Autodesk Inventor part; units mm, degrees
(part 3 of 13)
  spline S310 degree 3 poles (18.4407, 13.1537) (18.4407, 12.6177) (18.8752, 12.1831) (19.4112, 12.1831) knots 0 0 0 0 1 1 1 1
  line L939 (18.4407, 13.1537) -> (18.4407, 12.6177) construction
  line L940 (18.4407, 12.6177) -> (18.8752, 12.1831) construction
  line L941 (18.8752, 12.1831) -> (19.4112, 12.1831) construction
  spline S311 degree 3 poles (19.4112, 12.1831) (19.9472, 12.1831) (20.3818, 12.6177) (20.3818, 13.1537) knots 0 0 0 0 1 1 1 1
  line L942 (19.4112, 12.1831) -> (19.9472, 12.1831) construction
  line L943 (19.9472, 12.1831) -> (20.3818, 12.6177) construction
  line L944 (20.3818, 12.6177) -> (20.3818, 13.1537) construction
  spline S312 degree 3 poles (20.3818, 15.7078) (20.3818, 16.2438) (19.9472, 16.6783) (19.4112, 16.6783) knots 0 0 0 0 1 1 1 1
  line L945 (20.3818, 15.7078) -> (20.3818, 16.2438) construction
  line L946 (20.3818, 16.2438) -> (19.9472, 16.6783) construction
  line L947 (19.9472, 16.6783) -> (19.4112, 16.6783) construction
  spline S313 degree 3 poles (19.4112, 16.6783) (18.8752, 16.6783) (18.4407, 16.2438) (18.4407, 15.7078) knots 0 0 0 0 1 1 1 1
  line L948 (19.4112, 16.6783) -> (18.8752, 16.6783) construction
  line L949 (18.8752, 16.6783) -> (18.4407, 16.2438) construction
  line L950 (18.4407, 16.2438) -> (18.4407, 15.7078) construction
  spline S314 degree 3 poles (18.4407, 15.7078) (18.4407, 15.1718) (18.8752, 14.7372) (19.4112, 14.7372) knots 0 0 0 0 1 1 1 1
  line L951 (18.4407, 15.7078) -> (18.4407, 15.1718) construction
  line L952 (18.4407, 15.1718) -> (18.8752, 14.7372) construction
  line L953 (18.8752, 14.7372) -> (19.4112, 14.7372) construction
  spline S315 degree 3 poles (19.4112, 14.7372) (19.9472, 14.7372) (20.3818, 15.1718) (20.3818, 15.7078) knots 0 0 0 0 1 1 1 1
  line L954 (19.4112, 14.7372) -> (19.9472, 14.7372) construction
  line L955 (19.9472, 14.7372) -> (20.3818, 15.1718) construction
  line L956 (20.3818, 15.1718) -> (20.3818, 15.7078) construction
  spline S316 degree 3 poles (20.3818, 18.2619) (20.3818, 18.7979) (19.9472, 19.2324) (19.4112, 19.2324) knots 0 0 0 0 1 1 1 1
  line L957 (20.3818, 18.2619) -> (20.3818, 18.7979) construction
  line L958 (20.3818, 18.7979) -> (19.9472, 19.2324) construction
  line L959 (19.9472, 19.2324) -> (19.4112, 19.2324) construction
  spline S317 degree 3 poles (19.4112, 19.2324) (18.8752, 19.2324) (18.4407, 18.7979) (18.4407, 18.2619) knots 0 0 0 0 1 1 1 1
  line L960 (19.4112, 19.2324) -> (18.8752, 19.2324) construction
  line L961 (18.8752, 19.2324) -> (18.4407, 18.7979) construction
  line L962 (18.4407, 18.7979) -> (18.4407, 18.2619) construction
  spline S318 degree 3 poles (18.4407, 18.2619) (18.4407, 17.7259) (18.8752, 17.2914) (19.4112, 17.2914) knots 0 0 0 0 1 1 1 1
  line L963 (18.4407, 18.2619) -> (18.4407, 17.7259) construction
  line L964 (18.4407, 17.7259) -> (18.8752, 17.2914) construction
  line L965 (18.8752, 17.2914) -> (19.4112, 17.2914) construction
  spline S319 degree 3 poles (19.4112, 17.2914) (19.9472, 17.2914) (20.3818, 17.7259) (20.3818, 18.2619) knots 0 0 0 0 1 1 1 1
  line L966 (19.4112, 17.2914) -> (19.9472, 17.2914) construction
  line L967 (19.9472, 17.2914) -> (20.3818, 17.7259) construction
  line L968 (20.3818, 17.7259) -> (20.3818, 18.2619) construction
  spline S320 degree 3 poles (20.3818, 20.816) (20.3818, 21.352) (19.9472, 21.7866) (19.4112, 21.7866) knots 0 0 0 0 1 1 1 1
  line L969 (20.3818, 20.816) -> (20.3818, 21.352) construction
  line L970 (20.3818, 21.352) -> (19.9472, 21.7866) construction
  line L971 (19.9472, 21.7866) -> (19.4112, 21.7866) construction
  spline S321 degree 3 poles (19.4112, 21.7866) (18.8752, 21.7866) (18.4407, 21.352) (18.4407, 20.816) knots 0 0 0 0 1 1 1 1
  line L972 (19.4112, 21.7866) -> (18.8752, 21.7866) construction
  line L973 (18.8752, 21.7866) -> (18.4407, 21.352) construction
  line L974 (18.4407, 21.352) -> (18.4407, 20.816) construction
  spline S322 degree 3 poles (18.4407, 20.816) (18.4407, 20.28) (18.8752, 19.8455) (19.4112, 19.8455) knots 0 0 0 0 1 1 1 1
  line L975 (18.4407, 20.816) -> (18.4407, 20.28) construction
  line L976 (18.4407, 20.28) -> (18.8752, 19.8455) construction
  line L977 (18.8752, 19.8455) -> (19.4112, 19.8455) construction
  spline S323 degree 3 poles (19.4112, 19.8455) (19.9472, 19.8455) (20.3818, 20.28) (20.3818, 20.816) knots 0 0 0 0 1 1 1 1
  line L978 (19.4112, 19.8455) -> (19.9472, 19.8455) construction
  line L979 (19.9472, 19.8455) -> (20.3818, 20.28) construction
  line L980 (20.3818, 20.28) -> (20.3818, 20.816) construction
  line L981 (31.1601, 33.5866) -> (31.1601, 12.7705)
  line L982 (38.567, 33.7142) -> (38.567, 33.4588)
  line L983 (41.1212, 33.7142) -> (41.1212, 33.4588)
  line L984 (43.6753, 33.7142) -> (43.6753, 33.4588)
  line L985 (46.2294, 33.7142) -> (46.2294, 33.4588)
  line L986 (47.5064, 32.6927) -> (37.29, 32.6927)
  line L987 (47.5064, 34.4805) -> (37.29, 34.4805)
  line L988 (37.29, 16.6017) -> (34.7358, 16.6017)
  line L989 (36.0129, 15.8354) -> (36.0129, 15.58)
  line L990 (37.29, 17.368) -> (34.7358, 17.368)
  line L991 (36.0129, 18.3895) -> (36.0129, 18.1341)
  line L992 (37.29, 19.1558) -> (34.7358, 19.1558)
  line L993 (37.29, 19.9221) -> (34.7358, 19.9221)
  line L994 (37.29, 21.7099) -> (34.7358, 21.7099)
  line L995 (36.0129, 20.9436) -> (36.0129, 20.6882)
  line L996 (37.29, 22.4762) -> (34.7358, 22.4762)
  line L997 (36.0129, 23.4977) -> (36.0129, 23.2424)
  line L998 (37.29, 24.264) -> (34.7358, 24.264)
  line L999 (37.29, 25.0303) -> (34.7358, 25.0303)
  line L1000 (37.29, 26.8181) -> (34.7358, 26.8181)
  line L1001 (36.0129, 26.0518) -> (36.0129, 25.7965)
  line L1002 (37.29, 27.5844) -> (34.7358, 27.5844)
  line L1003 (36.0129, 28.606) -> (36.0129, 28.3506)
  line L1004 (37.29, 29.3723) -> (34.7358, 29.3723)
  line L1005 (37.29, 30.1386) -> (34.7358, 30.1386)
  line L1006 (36.0129, 31.1601) -> (36.0129, 30.9047)
  line L1007 (16.8571, 32.6927) -> (6.6406, 32.6927)
  line L1008 (10.4718, 33.7142) -> (10.4718, 33.4588)
  line L1009 (16.8571, 34.4805) -> (6.6406, 34.4805)
  line L1010 (13.0259, 33.7142) -> (13.0259, 33.4588)
  line L1011 (15.58, 33.7142) -> (15.58, 33.4588)
  line L1012 (7.9177, 33.7142) -> (7.9177, 33.4588)
  line L1013 (18.1341, 31.1601) -> (18.1341, 30.9047)
  line L1014 (16.8571, -0.5108) -> (6.6406, -0.5108)
  line L1015 (10.4718, 0.5108) -> (10.4718, 0.2554)
  line L1016 (16.8571, 1.2771) -> (6.6406, 1.2771)
  line L1017 (13.0259, 0.5108) -> (13.0259, 0.2554)
  line L1018 (15.58, 0.5108) -> (15.58, 0.2554)
  line L1019 (7.9177, 0.5108) -> (7.9177, 0.2554)
  line L1020 (19.4112, 2.0434) -> (16.8571, 2.0434)
  line L1021 (18.1341, 3.0649) -> (18.1341, 2.8095)
  line L1022 (19.4112, 3.8312) -> (16.8571, 3.8312)
  line L1023 (19.4112, 4.5975) -> (16.8571, 4.5975)
  line L1024 (19.4112, 6.3853) -> (16.8571, 6.3853)
  line L1025 (18.1341, 5.619) -> (18.1341, 5.3636)
  line L1026 (19.4112, 7.1516) -> (16.8571, 7.1516)
  line L1027 (19.4112, 8.9394) -> (16.8571, 8.9394)
  line L1028 (19.4112, 9.7057) -> (16.8571, 9.7057)
  line L1029 (18.1341, 8.1731) -> (18.1341, 7.9177)
  line L1030 (19.4112, 11.4935) -> (16.8571, 11.4935)
  line L1031 (18.1341, 10.7272) -> (18.1341, 10.4718)
  line L1032 (47.5064, -0.5108) -> (37.29, -0.5108)
  line L1033 (41.1212, 0.5108) -> (41.1212, 0.2554)
  line L1034 (47.5064, 1.2771) -> (37.29, 1.2771)
  line L1035 (43.6753, 0.5108) -> (43.6753, 0.2554)
  line L1036 (46.2294, 0.5108) -> (46.2294, 0.2554)
  line L1037 (38.567, 0.5108) -> (38.567, 0.2554)
  line L1038 (37.29, 2.0434) -> (34.7358, 2.0434)
  line L1039 (36.0129, 3.0649) -> (36.0129, 2.8095)
  line L1040 (37.29, 3.8312) -> (34.7358, 3.8312)
  line L1041 (37.29, 4.5975) -> (34.7358, 4.5975)
  line L1042 (37.29, 6.3853) -> (34.7358, 6.3853)
  line L1043 (36.0129, 5.619) -> (36.0129, 5.3636)
  line L1044 (37.29, 7.1516) -> (34.7358, 7.1516)
  line L1045 (36.0129, 8.1731) -> (36.0129, 7.9177)
  line L1046 (37.29, 8.9394) -> (34.7358, 8.9394)
  line L1047 (37.29, 9.7057) -> (34.7358, 9.7057)
  line L1048 (37.29, 11.4935) -> (34.7358, 11.4935)
  line L1049 (36.0129, 10.7272) -> (36.0129, 10.4718)
  line L1050 (37.29, 12.2598) -> (34.7358, 12.2598)
  line L1051 (36.0129, 13.2813) -> (36.0129, 13.0259)
  line L1052 (37.29, 14.0476) -> (34.7358, 14.0476)
  line L1053 (37.29, 14.8139) -> (34.7358, 14.8139)
  line L1054 (19.4112, 12.2598) -> (16.8571, 12.2598)
  line L1055 (18.1341, 13.2813) -> (18.1341, 13.0259)
  line L1056 (19.4112, 14.0476) -> (16.8571, 14.0476)
  line L1057 (19.4112, 14.8139) -> (16.8571, 14.8139)
  line L1058 (19.4112, 16.6017) -> (16.8571, 16.6017)
  line L1059 (18.1341, 15.8354) -> (18.1341, 15.58)
  line L1060 (19.4112, 17.368) -> (16.8571, 17.368)
  line L1061 (19.4112, 19.1558) -> (16.8571, 19.1558)
  line L1062 (19.4112, 19.9221) -> (16.8571, 19.9221)
  line L1063 (18.1341, 18.3895) -> (18.1341, 18.1341)
  line L1064 (19.4112, 21.7099) -> (16.8571, 21.7099)
  line L1065 (18.1341, 20.9436) -> (18.1341, 20.6882)
  line L1066 (19.4112, 22.4762) -> (16.8571, 22.4762)
  line L1067 (18.1341, 23.4977) -> (18.1341, 23.2424)
  line L1068 (19.4112, 24.264) -> (16.8571, 24.264)
  line L1069 (19.4112, 25.0303) -> (16.8571, 25.0303)
  line L1070 (19.4112, 26.8181) -> (16.8571, 26.8181)
  line L1071 (18.1341, 26.0518) -> (18.1341, 25.7965)
  line L1072 (19.4112, 27.5844) -> (16.8571, 27.5844)
  line L1073 (19.4112, 29.3723) -> (16.8571, 29.3723)
  line L1074 (19.4112, 30.1386) -> (16.8571, 30.1386)
  line L1075 (18.1341, 28.606) -> (18.1341, 28.3506)
  line L1076 (24.9026, 21.3779) -> (22.3485, 21.3779)
  line L1077 (23.6255, 22.3996) -> (23.6255, 22.1441)
  line L1078 (24.9026, 23.1657) -> (22.3485, 23.1657)
  line L1079 (24.9026, 23.932) -> (22.3485, 23.932)
  line L1080 (24.9026, 25.7198) -> (22.3485, 25.7198)
  line L1081 (23.6255, 24.9537) -> (23.6255, 24.6982)
  line L1082 (24.9026, 10.855) -> (22.3485, 10.855)
  line L1083 (24.9026, 12.6428) -> (22.3485, 12.6428)
  line L1084 (24.9026, 13.4091) -> (22.3485, 13.4091)
  line L1085 (23.6255, 11.8766) -> (23.6255, 11.6213)
  line L1086 (24.9026, 15.1969) -> (22.3485, 15.1969)
  spline S324 degree 3 poles (4.1377, 32.1817) (4.1377, 32.8447) (3.6002, 33.3822) (2.9373, 33.3822) knots 0 0 0 0 1 1 1 1
  line L1087 (4.1377, 32.1817) -> (4.1377, 32.8447) construction
  line L1088 (4.1377, 32.8447) -> (3.6002, 33.3822) construction
  line L1089 (3.6002, 33.3822) -> (2.9373, 33.3822) construction
  spline S325 degree 3 poles (2.9373, 33.3822) (2.2743, 33.3822) (1.7368, 32.8447) (1.7368, 32.1817) knots 0 0 0 0 1 1 1 1
  line L1090 (2.9373, 33.3822) -> (2.2743, 33.3822) construction
  line L1091 (2.2743, 33.3822) -> (1.7368, 32.8447) construction
  line L1092 (1.7368, 32.8447) -> (1.7368, 32.1817) construction
  spline S326 degree 3 poles (1.7368, 32.1817) (1.7368, 31.5188) (2.2743, 30.9813) (2.9373, 30.9813) knots 0 0 0 0 1 1 1 1
  line L1093 (1.7368, 32.1817) -> (1.7368, 31.5188) construction
  line L1094 (1.7368, 31.5188) -> (2.2743, 30.9813) construction
  line L1095 (2.2743, 30.9813) -> (2.9373, 30.9813) construction
  spline S327 degree 3 poles (2.9373, 30.9813) (3.6002, 30.9813) (4.1377, 31.5188) (4.1377, 32.1817) knots 0 0 0 0 1 1 1 1
  line L1096 (2.9373, 30.9813) -> (3.6002, 30.9813) construction
  line L1097 (3.6002, 30.9813) -> (4.1377, 31.5188) construction
  line L1098 (4.1377, 31.5188) -> (4.1377, 32.1817) construction
  spline S328 degree 3 poles (4.1377, 1.7878) (4.1377, 2.4507) (3.6002, 2.9882) (2.9373, 2.9882) knots 0 0 0 0 1 1 1 1
  line L1099 (4.1377, 1.7878) -> (4.1377, 2.4507) construction
  line L1100 (4.1377, 2.4507) -> (3.6002, 2.9882) construction
  line L1101 (3.6002, 2.9882) -> (2.9373, 2.9882) construction
  spline S329 degree 3 poles (2.9373, 2.9882) (2.2743, 2.9882) (1.7368, 2.4507) (1.7368, 1.7878) knots 0 0 0 0 1 1 1 1
  line L1102 (2.9373, 2.9882) -> (2.2743, 2.9882) construction
  line L1103 (2.2743, 2.9882) -> (1.7368, 2.4507) construction
  line L1104 (1.7368, 2.4507) -> (1.7368, 1.7878) construction
  spline S330 degree 3 poles (1.7368, 1.7878) (1.7368, 1.1249) (2.2743, 0.5874) (2.9373, 0.5874) knots 0 0 0 0 1 1 1 1
  line L1105 (1.7368, 1.7878) -> (1.7368, 1.1249) construction
  line L1106 (1.7368, 1.1249) -> (2.2743, 0.5874) construction
  line L1107 (2.2743, 0.5874) -> (2.9373, 0.5874) construction
  spline S331 degree 3 poles (2.9373, 0.5874) (3.6002, 0.5874) (4.1377, 1.1249) (4.1377, 1.7878) knots 0 0 0 0 1 1 1 1
  line L1108 (2.9373, 0.5874) -> (3.6002, 0.5874) construction
  line L1109 (3.6002, 0.5874) -> (4.1377, 1.1249) construction
  line L1110 (4.1377, 1.1249) -> (4.1377, 1.7878) construction
  spline S332 degree 3 poles (52.4103, 1.7878) (52.4103, 2.4507) (51.8729, 2.9882) (51.2099, 2.9882) knots 0 0 0 0 1 1 1 1
  line L1111 (52.4103, 1.7878) -> (52.4103, 2.4507) construction
  line L1112 (52.4103, 2.4507) -> (51.8729, 2.9882) construction
  line L1113 (51.8729, 2.9882) -> (51.2099, 2.9882) construction
  spline S333 degree 3 poles (51.2099, 2.9882) (50.5469, 2.9882) (50.0095, 2.4507) (50.0095, 1.7878) knots 0 0 0 0 1 1 1 1
  line L1114 (51.2099, 2.9882) -> (50.5469, 2.9882) construction
  line L1115 (50.5469, 2.9882) -> (50.0095, 2.4507) construction
  line L1116 (50.0095, 2.4507) -> (50.0095, 1.7878) construction
  spline S334 degree 3 poles (50.0095, 1.7878) (50.0095, 1.1249) (50.5469, 0.5874) (51.2099, 0.5874) knots 0 0 0 0 1 1 1 1
  line L1117 (50.0095, 1.7878) -> (50.0095, 1.1249) construction
  line L1118 (50.0095, 1.1249) -> (50.5469, 0.5874) construction
  line L1119 (50.5469, 0.5874) -> (51.2099, 0.5874) construction
  spline S335 degree 3 poles (51.2099, 0.5874) (51.8729, 0.5874) (52.4103, 1.1249) (52.4103, 1.7878) knots 0 0 0 0 1 1 1 1
  line L1120 (51.2099, 0.5874) -> (51.8729, 0.5874) construction
  line L1121 (51.8729, 0.5874) -> (52.4103, 1.1249) construction
  line L1122 (52.4103, 1.1249) -> (52.4103, 1.7878) construction
  spline S336 degree 3 poles (52.4103, 32.1817) (52.4103, 32.8447) (51.8729, 33.3822) (51.2099, 33.3822) knots 0 0 0 0 1 1 1 1
  line L1123 (52.4103, 32.1817) -> (52.4103, 32.8447) construction
  line L1124 (52.4103, 32.8447) -> (51.8729, 33.3822) construction
  line L1125 (51.8729, 33.3822) -> (51.2099, 33.3822) construction
  spline S337 degree 3 poles (51.2099, 33.3822) (50.5469, 33.3822) (50.0095, 32.8447) (50.0095, 32.1817) knots 0 0 0 0 1 1 1 1
  line L1126 (51.2099, 33.3822) -> (50.5469, 33.3822) construction
  line L1127 (50.5469, 33.3822) -> (50.0095, 32.8447) construction
  line L1128 (50.0095, 32.8447) -> (50.0095, 32.1817) construction
  spline S338 degree 3 poles (50.0095, 32.1817) (50.0095, 31.5188) (50.5469, 30.9813) (51.2099, 30.9813) knots 0 0 0 0 1 1 1 1
  line L1129 (50.0095, 32.1817) -> (50.0095, 31.5188) construction
  line L1130 (50.0095, 31.5188) -> (50.5469, 30.9813) construction
  line L1131 (50.5469, 30.9813) -> (51.2099, 30.9813) construction
  spline S339 degree 3 poles (51.2099, 30.9813) (51.8729, 30.9813) (52.4103, 31.5188) (52.4103, 32.1817) knots 0 0 0 0 1 1 1 1
  line L1132 (51.2099, 30.9813) -> (51.8729, 30.9813) construction
  line L1133 (51.8729, 30.9813) -> (52.4103, 31.5188) construction
  line L1134 (52.4103, 31.5188) -> (52.4103, 32.1817) construction
  spline S340 degree 3 poles (4.0865, 32.1817) (4.0865, 32.8164) (3.5719, 33.3312) (2.9373, 33.3312) knots 0 0 0 0 1 1 1 1
  line L1135 (4.0865, 32.1817) -> (4.0865, 32.8164) construction
  line L1136 (4.0865, 32.8164) -> (3.5719, 33.3312) construction
  line L1137 (3.5719, 33.3312) -> (2.9373, 33.3312) construction
  spline S341 degree 3 poles (2.9373, 33.3312) (2.3026, 33.3312) (1.7878, 32.8164) (1.7878, 32.1817) knots 0 0 0 0 1 1 1 1
  line L1138 (2.9373, 33.3312) -> (2.3026, 33.3312) construction
  line L1139 (2.3026, 33.3312) -> (1.7878, 32.8164) construction
  line L1140 (1.7878, 32.8164) -> (1.7878, 32.1817) construction
  spline S342 degree 3 poles (1.7878, 32.1817) (1.7878, 31.5471) (2.3026, 31.0325) (2.9373, 31.0325) knots 0 0 0 0 1 1 1 1
  line L1141 (1.7878, 32.1817) -> (1.7878, 31.5471) construction
  line L1142 (1.7878, 31.5471) -> (2.3026, 31.0325) construction
  line L1143 (2.3026, 31.0325) -> (2.9373, 31.0325) construction
  spline S343 degree 3 poles (2.9373, 31.0325) (3.5719, 31.0325) (4.0865, 31.5471) (4.0865, 32.1817) knots 0 0 0 0 1 1 1 1
  line L1144 (2.9373, 31.0325) -> (3.5719, 31.0325) construction
  line L1145 (3.5719, 31.0325) -> (4.0865, 31.5471) construction
  line L1146 (4.0865, 31.5471) -> (4.0865, 32.1817) construction
  spline S344 degree 3 poles (4.0865, 1.7878) (4.0865, 2.4225) (3.5719, 2.9373) (2.9373, 2.9373) knots 0 0 0 0 1 1 1 1
  line L1147 (4.0865, 1.7878) -> (4.0865, 2.4225) construction
  line L1148 (4.0865, 2.4225) -> (3.5719, 2.9373) construction
  line L1149 (3.5719, 2.9373) -> (2.9373, 2.9373) construction
  spline S345 degree 3 poles (2.9373, 2.9373) (2.3026, 2.9373) (1.7878, 2.4225) (1.7878, 1.7878) knots 0 0 0 0 1 1 1 1
  line L1150 (2.9373, 2.9373) -> (2.3026, 2.9373) construction
  line L1151 (2.3026, 2.9373) -> (1.7878, 2.4225) construction
  line L1152 (1.7878, 2.4225) -> (1.7878, 1.7878) construction
  spline S346 degree 3 poles (1.7878, 1.7878) (1.7878, 1.1532) (2.3026, 0.6385) (2.9373, 0.6385) knots 0 0 0 0 1 1 1 1
  line L1153 (1.7878, 1.7878) -> (1.7878, 1.1532) construction
  line L1154 (1.7878, 1.1532) -> (2.3026, 0.6385) construction
  line L1155 (2.3026, 0.6385) -> (2.9373, 0.6385) construction
  spline S347 degree 3 poles (2.9373, 0.6385) (3.5719, 0.6385) (4.0865, 1.1532) (4.0865, 1.7878) knots 0 0 0 0 1 1 1 1
  line L1156 (2.9373, 0.6385) -> (3.5719, 0.6385) construction
  line L1157 (3.5719, 0.6385) -> (4.0865, 1.1532) construction
  line L1158 (4.0865, 1.1532) -> (4.0865, 1.7878) construction
  spline S348 degree 3 poles (52.3592, 1.7878) (52.3592, 2.4225) (51.8445, 2.9373) (51.2099, 2.9373) knots 0 0 0 0 1 1 1 1
  line L1159 (52.3592, 1.7878) -> (52.3592, 2.4225) construction
  line L1160 (52.3592, 2.4225) -> (51.8445, 2.9373) construction
  line L1161 (51.8445, 2.9373) -> (51.2099, 2.9373) construction
  spline S349 degree 3 poles (51.2099, 2.9373) (50.5753, 2.9373) (50.0605, 2.4225) (50.0605, 1.7878) knots 0 0 0 0 1 1 1 1
  line L1162 (51.2099, 2.9373) -> (50.5753, 2.9373) construction
  line L1163 (50.5753, 2.9373) -> (50.0605, 2.4225) construction
  line L1164 (50.0605, 2.4225) -> (50.0605, 1.7878) construction
  spline S350 degree 3 poles (50.0605, 1.7878) (50.0605, 1.1532) (50.5753, 0.6385) (51.2099, 0.6385) knots 0 0 0 0 1 1 1 1
  line L1165 (50.0605, 1.7878) -> (50.0605, 1.1532) construction
  line L1166 (50.0605, 1.1532) -> (50.5753, 0.6385) construction
  line L1167 (50.5753, 0.6385) -> (51.2099, 0.6385) construction
  spline S351 degree 3 poles (51.2099, 0.6385) (51.8445, 0.6385) (52.3592, 1.1532) (52.3592, 1.7878) knots 0 0 0 0 1 1 1 1
  line L1168 (51.2099, 0.6385) -> (51.8445, 0.6385) construction
  line L1169 (51.8445, 0.6385) -> (52.3592, 1.1532) construction
  line L1170 (52.3592, 1.1532) -> (52.3592, 1.7878) construction
  spline S352 degree 3 poles (52.3592, 32.1817) (52.3592, 32.8164) (51.8445, 33.3312) (51.2099, 33.3312) knots 0 0 0 0 1 1 1 1
  line L1171 (52.3592, 32.1817) -> (52.3592, 32.8164) construction
  line L1172 (52.3592, 32.8164) -> (51.8445, 33.3312) construction
  line L1173 (51.8445, 33.3312) -> (51.2099, 33.3312) construction
  spline S353 degree 3 poles (51.2099, 33.3312) (50.5753, 33.3312) (50.0605, 32.8164) (50.0605, 32.1817) knots 0 0 0 0 1 1 1 1
  line L1174 (51.2099, 33.3312) -> (50.5753, 33.3312) construction
  line L1175 (50.5753, 33.3312) -> (50.0605, 32.8164) construction
  line L1176 (50.0605, 32.8164) -> (50.0605, 32.1817) construction
  spline S354 degree 3 poles (50.0605, 32.1817) (50.0605, 31.5471) (50.5753, 31.0325) (51.2099, 31.0325) knots 0 0 0 0 1 1 1 1
  line L1177 (50.0605, 32.1817) -> (50.0605, 31.5471) construction
  line L1178 (50.0605, 31.5471) -> (50.5753, 31.0325) construction
  line L1179 (50.5753, 31.0325) -> (51.2099, 31.0325) construction
  spline S355 degree 3 poles (51.2099, 31.0325) (51.8445, 31.0325) (52.3592, 31.5471) (52.3592, 32.1817) knots 0 0 0 0 1 1 1 1
  line L1180 (51.2099, 31.0325) -> (51.8445, 31.0325) construction
  line L1181 (51.8445, 31.0325) -> (52.3592, 31.5471) construction
  line L1182 (52.3592, 31.5471) -> (52.3592, 32.1817) construction
  spline S356 degree 3 poles (9.6418, 33.5866) (9.6418, 33.8334) (9.4415, 34.0334) (9.1948, 34.0334) knots 0 0 0 0 1 1 1 1
  line L1183 (9.6418, 33.5866) -> (9.6418, 33.8334) construction
  line L1184 (9.6418, 33.8334) -> (9.4415, 34.0334) construction
  line L1185 (9.4415, 34.0334) -> (9.1948, 34.0334) construction
  spline S357 degree 3 poles (9.1948, 34.0334) (8.948, 34.0334) (8.7479, 33.8334) (8.7479, 33.5866) knots 0 0 0 0 1 1 1 1
  line L1186 (9.1948, 34.0334) -> (8.948, 34.0334) construction
  line L1187 (8.948, 34.0334) -> (8.7479, 33.8334) construction
  line L1188 (8.7479, 33.8334) -> (8.7479, 33.5866) construction
  spline S358 degree 3 poles (8.7479, 33.5866) (8.7479, 33.3398) (8.948, 33.1395) (9.1948, 33.1395) knots 0 0 0 0 1 1 1 1
  line L1189 (8.7479, 33.5866) -> (8.7479, 33.3398) construction
  line L1190 (8.7479, 33.3398) -> (8.948, 33.1395) construction
  line L1191 (8.948, 33.1395) -> (9.1948, 33.1395) construction
  spline S359 degree 3 poles (9.1948, 33.1395) (9.4415, 33.1395) (9.6418, 33.3398) (9.6418, 33.5866) knots 0 0 0 0 1 1 1 1
  line L1192 (9.1948, 33.1395) -> (9.4415, 33.1395) construction
  line L1193 (9.4415, 33.1395) -> (9.6418, 33.3398) construction
  line L1194 (9.6418, 33.3398) -> (9.6418, 33.5866) construction
  spline S360 degree 3 poles (12.1959, 33.5866) (12.1959, 33.8334) (11.9957, 34.0334) (11.7489, 34.0334) knots 0 0 0 0 1 1 1 1
  line L1195 (12.1959, 33.5866) -> (12.1959, 33.8334) construction
  line L1196 (12.1959, 33.8334) -> (11.9957, 34.0334) construction
  line L1197 (11.9957, 34.0334) -> (11.7489, 34.0334) construction
  spline S361 degree 3 poles (11.7489, 34.0334) (11.5021, 34.0334) (11.302, 33.8334) (11.302, 33.5866) knots 0 0 0 0 1 1 1 1
  line L1198 (11.7489, 34.0334) -> (11.5021, 34.0334) construction
  line L1199 (11.5021, 34.0334) -> (11.302, 33.8334) construction
  line L1200 (11.302, 33.8334) -> (11.302, 33.5866) construction
  spline S362 degree 3 poles (11.302, 33.5866) (11.302, 33.3398) (11.5021, 33.1395) (11.7489, 33.1395) knots 0 0 0 0 1 1 1 1
  line L1201 (11.302, 33.5866) -> (11.302, 33.3398) construction
  line L1202 (11.302, 33.3398) -> (11.5021, 33.1395) construction
  line L1203 (11.5021, 33.1395) -> (11.7489, 33.1395) construction
  spline S363 degree 3 poles (11.7489, 33.1395) (11.9957, 33.1395) (12.1959, 33.3398) (12.1959, 33.5866) knots 0 0 0 0 1 1 1 1
  line L1204 (11.7489, 33.1395) -> (11.9957, 33.1395) construction
  line L1205 (11.9957, 33.1395) -> (12.1959, 33.3398) construction
  line L1206 (12.1959, 33.3398) -> (12.1959, 33.5866) construction
  spline S364 degree 3 poles (14.75, 33.5866) (14.75, 33.8334) (14.5498, 34.0334) (14.303, 34.0334) knots 0 0 0 0 1 1 1 1
  line L1207 (14.75, 33.5866) -> (14.75, 33.8334) construction
  line L1208 (14.75, 33.8334) -> (14.5498, 34.0334) construction
  line L1209 (14.5498, 34.0334) -> (14.303, 34.0334) construction
  spline S365 degree 3 poles (14.303, 34.0334) (14.0562, 34.0334) (13.8561, 33.8334) (13.8561, 33.5866) knots 0 0 0 0 1 1 1 1
  line L1210 (14.303, 34.0334) -> (14.0562, 34.0334) construction
  line L1211 (14.0562, 34.0334) -> (13.8561, 33.8334) construction
  line L1212 (13.8561, 33.8334) -> (13.8561, 33.5866) construction
  spline S366 degree 3 poles (13.8561, 33.5866) (13.8561, 33.3398) (14.0562, 33.1395) (14.303, 33.1395) knots 0 0 0 0 1 1 1 1
  line L1213 (13.8561, 33.5866) -> (13.8561, 33.3398) construction
  line L1214 (13.8561, 33.3398) -> (14.0562, 33.1395) construction
  line L1215 (14.0562, 33.1395) -> (14.303, 33.1395) construction
  spline S367 degree 3 poles (14.303, 33.1395) (14.5498, 33.1395) (14.75, 33.3398) (14.75, 33.5866) knots 0 0 0 0 1 1 1 1
  line L1216 (14.303, 33.1395) -> (14.5498, 33.1395) construction
  line L1217 (14.5498, 33.1395) -> (14.75, 33.3398) construction
  line L1218 (14.75, 33.3398) -> (14.75, 33.5866) construction
  spline S368 degree 3 poles (17.3041, 23.3701) (17.3041, 23.6169) (17.1039, 23.817) (16.8571, 23.817) knots 0 0 0 0 1 1 1 1
  line L1219 (17.3041, 23.3701) -> (17.3041, 23.6169) construction
  line L1220 (17.3041, 23.6169) -> (17.1039, 23.817) construction
  line L1221 (17.1039, 23.817) -> (16.8571, 23.817) construction
  spline S369 degree 3 poles (16.8571, 23.817) (16.6103, 23.817) (16.4102, 23.6169) (16.4102, 23.3701) knots 0 0 0 0 1 1 1 1
  line L1222 (16.8571, 23.817) -> (16.6103, 23.817) construction
  line L1223 (16.6103, 23.817) -> (16.4102, 23.6169) construction
  line L1224 (16.4102, 23.6169) -> (16.4102, 23.3701) construction
  spline S370 degree 3 poles (16.4102, 23.3701) (16.4102, 23.1233) (16.6103, 22.9231) (16.8571, 22.9231) knots 0 0 0 0 1 1 1 1
  line L1225 (16.4102, 23.3701) -> (16.4102, 23.1233) construction
  line L1226 (16.4102, 23.1233) -> (16.6103, 22.9231) construction
  line L1227 (16.6103, 22.9231) -> (16.8571, 22.9231) construction
  spline S371 degree 3 poles (16.8571, 22.9231) (17.1039, 22.9231) (17.3041, 23.1233) (17.3041, 23.3701) knots 0 0 0 0 1 1 1 1
  line L1228 (16.8571, 22.9231) -> (17.1039, 22.9231) construction
  line L1229 (17.1039, 22.9231) -> (17.3041, 23.1233) construction
  line L1230 (17.3041, 23.1233) -> (17.3041, 23.3701) construction
  spline S372 degree 3 poles (22.7955, 22.2718) (22.7955, 22.5186) (22.5952, 22.7188) (22.3485, 22.7188) knots 0 0 0 0 1 1 1 1
  line L1231 (22.7955, 22.2718) -> (22.7955, 22.5186) construction
  line L1232 (22.7955, 22.5186) -> (22.5952, 22.7188) construction
  line L1233 (22.5952, 22.7188) -> (22.3485, 22.7188) construction
  spline S373 degree 3 poles (22.3485, 22.7188) (22.1017, 22.7188) (21.9014, 22.5186) (21.9014, 22.2718) knots 0 0 0 0 1 1 1 1
  line L1234 (22.3485, 22.7188) -> (22.1017, 22.7188) construction
  line L1235 (22.1017, 22.7188) -> (21.9014, 22.5186) construction
  line L1236 (21.9014, 22.5186) -> (21.9014, 22.2718) construction
  spline S374 degree 3 poles (21.9014, 22.2718) (21.9014, 22.025) (22.1017, 21.8248) (22.3485, 21.8248) knots 0 0 0 0 1 1 1 1
  line L1237 (21.9014, 22.2718) -> (21.9014, 22.025) construction
  line L1238 (21.9014, 22.025) -> (22.1017, 21.8248) construction
  line L1239 (22.1017, 21.8248) -> (22.3485, 21.8248) construction
  spline S375 degree 3 poles (22.3485, 21.8248) (22.5952, 21.8248) (22.7955, 22.025) (22.7955, 22.2718) knots 0 0 0 0 1 1 1 1
  line L1240 (22.3485, 21.8248) -> (22.5952, 21.8248) construction
  line L1241 (22.5952, 21.8248) -> (22.7955, 22.025) construction
  line L1242 (22.7955, 22.025) -> (22.7955, 22.2718) construction
  spline S376 degree 3 poles (25.3496, 22.2718) (25.3496, 22.5186) (25.1494, 22.7188) (24.9026, 22.7188) knots 0 0 0 0 1 1 1 1
  line L1243 (25.3496, 22.2718) -> (25.3496, 22.5186) construction
  line L1244 (25.3496, 22.5186) -> (25.1494, 22.7188) construction
  line L1245 (25.1494, 22.7188) -> (24.9026, 22.7188) construction
  spline S377 degree 3 poles (24.9026, 22.7188) (24.6558, 22.7188) (24.4555, 22.5186) (24.4555, 22.2718) knots 0 0 0 0 1 1 1 1
  line L1246 (24.9026, 22.7188) -> (24.6558, 22.7188) construction
  line L1247 (24.6558, 22.7188) -> (24.4555, 22.5186) construction
  line L1248 (24.4555, 22.5186) -> (24.4555, 22.2718) construction
  spline S378 degree 3 poles (24.4555, 22.2718) (24.4555, 22.025) (24.6558, 21.8248) (24.9026, 21.8248) knots 0 0 0 0 1 1 1 1
  line L1249 (24.4555, 22.2718) -> (24.4555, 22.025) construction
  line L1250 (24.4555, 22.025) -> (24.6558, 21.8248) construction
  line L1251 (24.6558, 21.8248) -> (24.9026, 21.8248) construction
  spline S379 degree 3 poles (24.9026, 21.8248) (25.1494, 21.8248) (25.3496, 22.025) (25.3496, 22.2718) knots 0 0 0 0 1 1 1 1
  line L1252 (24.9026, 21.8248) -> (25.1494, 21.8248) construction
  line L1253 (25.1494, 21.8248) -> (25.3496, 22.025) construction
  line L1254 (25.3496, 22.025) -> (25.3496, 22.2718) construction
  spline S380 degree 3 poles (22.7955, 24.8259) (22.7955, 25.0727) (22.5952, 25.2729) (22.3485, 25.2729) knots 0 0 0 0 1 1 1 1
  line L1255 (22.7955, 24.8259) -> (22.7955, 25.0727) construction
  line L1256 (22.7955, 25.0727) -> (22.5952, 25.2729) construction
  line L1257 (22.5952, 25.2729) -> (22.3485, 25.2729) construction
  spline S381 degree 3 poles (22.3485, 25.2729) (22.1017, 25.2729) (21.9014, 25.0727) (21.9014, 24.8259) knots 0 0 0 0 1 1 1 1
  line L1258 (22.3485, 25.2729) -> (22.1017, 25.2729) construction
  line L1259 (22.1017, 25.2729) -> (21.9014, 25.0727) construction
  line L1260 (21.9014, 25.0727) -> (21.9014, 24.8259) construction
  spline S382 degree 3 poles (21.9014, 24.8259) (21.9014, 24.5792) (22.1017, 24.3789) (22.3485, 24.3789) knots 0 0 0 0 1 1 1 1
  line L1261 (21.9014, 24.8259) -> (21.9014, 24.5792) construction
  line L1262 (21.9014, 24.5792) -> (22.1017, 24.3789) construction
  line L1263 (22.1017, 24.3789) -> (22.3485, 24.3789) construction
  spline S383 degree 3 poles (22.3485, 24.3789) (22.5952, 24.3789) (22.7955, 24.5792) (22.7955, 24.8259) knots 0 0 0 0 1 1 1 1
  line L1264 (22.3485, 24.3789) -> (22.5952, 24.3789) construction
  line L1265 (22.5952, 24.3789) -> (22.7955, 24.5792) construction
  line L1266 (22.7955, 24.5792) -> (22.7955, 24.8259) construction
  spline S384 degree 3 poles (25.3496, 24.8259) (25.3496, 25.0727) (25.1494, 25.2729) (24.9026, 25.2729) knots 0 0 0 0 1 1 1 1
  line L1267 (25.3496, 24.8259) -> (25.3496, 25.0727) construction
  line L1268 (25.3496, 25.0727) -> (25.1494, 25.2729) construction
  line L1269 (25.1494, 25.2729) -> (24.9026, 25.2729) construction
  spline S385 degree 3 poles (24.9026, 25.2729) (24.6558, 25.2729) (24.4555, 25.0727) (24.4555, 24.8259) knots 0 0 0 0 1 1 1 1
  line L1270 (24.9026, 25.2729) -> (24.6558, 25.2729) construction
  line L1271 (24.6558, 25.2729) -> (24.4555, 25.0727) construction
  line L1272 (24.4555, 25.0727) -> (24.4555, 24.8259) construction
  spline S386 degree 3 poles (24.4555, 24.8259) (24.4555, 24.5792) (24.6558, 24.3789) (24.9026, 24.3789) knots 0 0 0 0 1 1 1 1
  line L1273 (24.4555, 24.8259) -> (24.4555, 24.5792) construction
  line L1274 (24.4555, 24.5792) -> (24.6558, 24.3789) construction
  line L1275 (24.6558, 24.3789) -> (24.9026, 24.3789) construction
  spline S387 degree 3 poles (24.9026, 24.3789) (25.1494, 24.3789) (25.3496, 24.5792) (25.3496, 24.8259) knots 0 0 0 0 1 1 1 1
  line L1276 (24.9026, 24.3789) -> (25.1494, 24.3789) construction
  line L1277 (25.1494, 24.3789) -> (25.3496, 24.5792) construction
  line L1278 (25.3496, 24.5792) -> (25.3496, 24.8259) construction
  spline S388 degree 3 poles (19.8582, 23.3701) (19.8582, 23.6169) (19.658, 23.817) (19.4112, 23.817) knots 0 0 0 0 1 1 1 1
  line L1279 (19.8582, 23.3701) -> (19.8582, 23.6169) construction
  line L1280 (19.8582, 23.6169) -> (19.658, 23.817) construction
  line L1281 (19.658, 23.817) -> (19.4112, 23.817) construction
  spline S389 degree 3 poles (19.4112, 23.817) (19.1644, 23.817) (18.9643, 23.6169) (18.9643, 23.3701) knots 0 0 0 0 1 1 1 1
  line L1282 (19.4112, 23.817) -> (19.1644, 23.817) construction
  line L1283 (19.1644, 23.817) -> (18.9643, 23.6169) construction
  line L1284 (18.9643, 23.6169) -> (18.9643, 23.3701) construction
  spline S390 degree 3 poles (18.9643, 23.3701) (18.9643, 23.1233) (19.1644, 22.9231) (19.4112, 22.9231) knots 0 0 0 0 1 1 1 1
  line L1285 (18.9643, 23.3701) -> (18.9643, 23.1233) construction
  line L1286 (18.9643, 23.1233) -> (19.1644, 22.9231) construction
  line L1287 (19.1644, 22.9231) -> (19.4112, 22.9231) construction
  spline S391 degree 3 poles (19.4112, 22.9231) (19.658, 22.9231) (19.8582, 23.1233) (19.8582, 23.3701) knots 0 0 0 0 1 1 1 1
  line L1288 (19.4112, 22.9231) -> (19.658, 22.9231) construction
  line L1289 (19.658, 22.9231) -> (19.8582, 23.1233) construction
  line L1290 (19.8582, 23.1233) -> (19.8582, 23.3701) construction
  spline S392 degree 3 poles (19.8582, 25.9242) (19.8582, 26.171) (19.658, 26.3711) (19.4112, 26.3711) knots 0 0 0 0 1 1 1 1
  line L1291 (19.8582, 25.9242) -> (19.8582, 26.171) construction
  line L1292 (19.8582, 26.171) -> (19.658, 26.3711) construction
  line L1293 (19.658, 26.3711) -> (19.4112, 26.3711) construction
  spline S393 degree 3 poles (19.4112, 26.3711) (19.1644, 26.3711) (18.9643, 26.171) (18.9643, 25.9242) knots 0 0 0 0 1 1 1 1
  line L1294 (19.4112, 26.3711) -> (19.1644, 26.3711) construction
  line L1295 (19.1644, 26.3711) -> (18.9643, 26.171) construction
  line L1296 (18.9643, 26.171) -> (18.9643, 25.9242) construction
  spline S394 degree 3 poles (18.9643, 25.9242) (18.9643, 25.6775) (19.1644, 25.4772) (19.4112, 25.4772) knots 0 0 0 0 1 1 1 1
  line L1297 (18.9643, 25.9242) -> (18.9643, 25.6775) construction
  line L1298 (18.9643, 25.6775) -> (19.1644, 25.4772) construction
  line L1299 (19.1644, 25.4772) -> (19.4112, 25.4772) construction
  spline S395 degree 3 poles (19.4112, 25.4772) (19.658, 25.4772) (19.8582, 25.6775) (19.8582, 25.9242) knots 0 0 0 0 1 1 1 1
  line L1300 (19.4112, 25.4772) -> (19.658, 25.4772) construction
  line L1301 (19.658, 25.4772) -> (19.8582, 25.6775) construction
  line L1302 (19.8582, 25.6775) -> (19.8582, 25.9242) construction
  spline S396 degree 3 poles (19.8582, 28.4784) (19.8582, 28.7251) (19.658, 28.9252) (19.4112, 28.9252) knots 0 0 0 0 1 1 1 1
  line L1303 (19.8582, 28.4784) -> (19.8582, 28.7251) construction
  line L1304 (19.8582, 28.7251) -> (19.658, 28.9252) construction
  line L1305 (19.658, 28.9252) -> (19.4112, 28.9252) construction
  spline S397 degree 3 poles (19.4112, 28.9252) (19.1644, 28.9252) (18.9643, 28.7251) (18.9643, 28.4784) knots 0 0 0 0 1 1 1 1
  line L1306 (19.4112, 28.9252) -> (19.1644, 28.9252) construction
  line L1307 (19.1644, 28.9252) -> (18.9643, 28.7251) construction
  line L1308 (18.9643, 28.7251) -> (18.9643, 28.4784) construction
  spline S398 degree 3 poles (18.9643, 28.4784) (18.9643, 28.2316) (19.1644, 28.0313) (19.4112, 28.0313) knots 0 0 0 0 1 1 1 1
  line L1309 (18.9643, 28.4784) -> (18.9643, 28.2316) construction
  line L1310 (18.9643, 28.2316) -> (19.1644, 28.0313) construction
  line L1311 (19.1644, 28.0313) -> (19.4112, 28.0313) construction
  spline S399 degree 3 poles (19.4112, 28.0313) (19.658, 28.0313) (19.8582, 28.2316) (19.8582, 28.4784) knots 0 0 0 0 1 1 1 1
  line L1312 (19.4112, 28.0313) -> (19.658, 28.0313) construction
  line L1313 (19.658, 28.0313) -> (19.8582, 28.2316) construction
  line L1314 (19.8582, 28.2316) -> (19.8582, 28.4784) construction
  spline S400 degree 3 poles (19.8582, 31.0325) (19.8582, 31.2793) (19.658, 31.4793) (19.4112, 31.4793) knots 0 0 0 0 1 1 1 1
  line L1315 (19.8582, 31.0325) -> (19.8582, 31.2793) construction
  line L1316 (19.8582, 31.2793) -> (19.658, 31.4793) construction
  line L1317 (19.658, 31.4793) -> (19.4112, 31.4793) construction
  spline S401 degree 3 poles (19.4112, 31.4793) (19.1644, 31.4793) (18.9643, 31.2793) (18.9643, 31.0325) knots 0 0 0 0 1 1 1 1
  line L1318 (19.4112, 31.4793) -> (19.1644, 31.4793) construction
  line L1319 (19.1644, 31.4793) -> (18.9643, 31.2793) construction
  line L1320 (18.9643, 31.2793) -> (18.9643, 31.0325) construction
  spline S402 degree 3 poles (18.9643, 31.0325) (18.9643, 30.7857) (19.1644, 30.5854) (19.4112, 30.5854) knots 0 0 0 0 1 1 1 1
  line L1321 (18.9643, 31.0325) -> (18.9643, 30.7857) construction
  line L1322 (18.9643, 30.7857) -> (19.1644, 30.5854) construction
  line L1323 (19.1644, 30.5854) -> (19.4112, 30.5854) construction
  spline S403 degree 3 poles (19.4112, 30.5854) (19.658, 30.5854) (19.8582, 30.7857) (19.8582, 31.0325) knots 0 0 0 0 1 1 1 1
  line L1324 (19.4112, 30.5854) -> (19.658, 30.5854) construction
  line L1325 (19.658, 30.5854) -> (19.8582, 30.7857) construction
  line L1326 (19.8582, 30.7857) -> (19.8582, 31.0325) construction
  spline S404 degree 3 poles (17.3041, 25.9242) (17.3041, 26.171) (17.1039, 26.3711) (16.8571, 26.3711) knots 0 0 0 0 1 1 1 1
  line L1327 (17.3041, 25.9242) -> (17.3041, 26.171) construction
  line L1328 (17.3041, 26.171) -> (17.1039, 26.3711) construction
  line L1329 (17.1039, 26.3711) -> (16.8571, 26.3711) construction
  spline S405 degree 3 poles (16.8571, 26.3711) (16.6103, 26.3711) (16.4102, 26.171) (16.4102, 25.9242) knots 0 0 0 0 1 1 1 1
  line L1330 (16.8571, 26.3711) -> (16.6103, 26.3711) construction
  line L1331 (16.6103, 26.3711) -> (16.4102, 26.171) construction
  line L1332 (16.4102, 26.171) -> (16.4102, 25.9242) construction
  spline S406 degree 3 poles (16.4102, 25.9242) (16.4102, 25.6775) (16.6103, 25.4772) (16.8571, 25.4772) knots 0 0 0 0 1 1 1 1
  line L1333 (16.4102, 25.9242) -> (16.4102, 25.6775) construction
  line L1334 (16.4102, 25.6775) -> (16.6103, 25.4772) construction
  line L1335 (16.6103, 25.4772) -> (16.8571, 25.4772) construction
  spline S407 degree 3 poles (16.8571, 25.4772) (17.1039, 25.4772) (17.3041, 25.6775) (17.3041, 25.9242) knots 0 0 0 0 1 1 1 1
  line L1336 (16.8571, 25.4772) -> (17.1039, 25.4772) construction
  line L1337 (17.1039, 25.4772) -> (17.3041, 25.6775) construction
  line L1338 (17.3041, 25.6775) -> (17.3041, 25.9242) construction
  spline S408 degree 3 poles (17.3041, 28.4784) (17.3041, 28.7251) (17.1039, 28.9252) (16.8571, 28.9252) knots 0 0 0 0 1 1 1 1
  line L1339 (17.3041, 28.4784) -> (17.3041, 28.7251) construction
  line L1340 (17.3041, 28.7251) -> (17.1039, 28.9252) construction
  line L1341 (17.1039, 28.9252) -> (16.8571, 28.9252) construction
  spline S409 degree 3 poles (16.8571, 28.9252) (16.6103, 28.9252) (16.4102, 28.7251) (16.4102, 28.4784) knots 0 0 0 0 1 1 1 1
  line L1342 (16.8571, 28.9252) -> (16.6103, 28.9252) construction
  line L1343 (16.6103, 28.9252) -> (16.4102, 28.7251) construction
  line L1344 (16.4102, 28.7251) -> (16.4102, 28.4784) construction
  spline S410 degree 3 poles (16.4102, 28.4784) (16.4102, 28.2316) (16.6103, 28.0313) (16.8571, 28.0313) knots 0 0 0 0 1 1 1 1
  line L1345 (16.4102, 28.4784) -> (16.4102, 28.2316) construction
  line L1346 (16.4102, 28.2316) -> (16.6103, 28.0313) construction
  line L1347 (16.6103, 28.0313) -> (16.8571, 28.0313) construction
  spline S411 degree 3 poles (16.8571, 28.0313) (17.1039, 28.0313) (17.3041, 28.2316) (17.3041, 28.4784) knots 0 0 0 0 1 1 1 1
  line L1348 (16.8571, 28.0313) -> (17.1039, 28.0313) construction
  line L1349 (17.1039, 28.0313) -> (17.3041, 28.2316) construction
  line L1350 (17.3041, 28.2316) -> (17.3041, 28.4784) construction
  spline S412 degree 3 poles (17.3041, 31.0325) (17.3041, 31.2793) (17.1039, 31.4793) (16.8571, 31.4793) knots 0 0 0 0 1 1 1 1
  line L1351 (17.3041, 31.0325) -> (17.3041, 31.2793) construction
  line L1352 (17.3041, 31.2793) -> (17.1039, 31.4793) construction
  line L1353 (17.1039, 31.4793) -> (16.8571, 31.4793) construction
  spline S413 degree 3 poles (16.8571, 31.4793) (16.6103, 31.4793) (16.4102, 31.2793) (16.4102, 31.0325) knots 0 0 0 0 1 1 1 1
  line L1354 (16.8571, 31.4793) -> (16.6103, 31.4793) construction
  line L1355 (16.6103, 31.4793) -> (16.4102, 31.2793) construction
  line L1356 (16.4102, 31.2793) -> (16.4102, 31.0325) construction
  spline S414 degree 3 poles (16.4102, 31.0325) (16.4102, 30.7857) (16.6103, 30.5854) (16.8571, 30.5854) knots 0 0 0 0 1 1 1 1
  line L1357 (16.4102, 31.0325) -> (16.4102, 30.7857) construction
  line L1358 (16.4102, 30.7857) -> (16.6103, 30.5854) construction
  line L1359 (16.6103, 30.5854) -> (16.8571, 30.5854) construction
  spline S415 degree 3 poles (16.8571, 30.5854) (17.1039, 30.5854) (17.3041, 30.7857) (17.3041, 31.0325) knots 0 0 0 0 1 1 1 1
  line L1360 (16.8571, 30.5854) -> (17.1039, 30.5854) construction
  line L1361 (17.1039, 30.5854) -> (17.3041, 30.7857) construction
  line L1362 (17.3041, 30.7857) -> (17.3041, 31.0325) construction
  spline S416 degree 3 poles (37.737, 33.5866) (37.737, 33.8334) (37.5369, 34.0334) (37.29, 34.0334) knots 0 0 0 0 1 1 1 1
  line L1363 (37.737, 33.5866) -> (37.737, 33.8334) construction
  line L1364 (37.737, 33.8334) -> (37.5369, 34.0334) construction
  line L1365 (37.5369, 34.0334) -> (37.29, 34.0334) construction
  spline S417 degree 3 poles (37.29, 34.0334) (37.0431, 34.0334) (36.843, 33.8334) (36.843, 33.5866) knots 0 0 0 0 1 1 1 1
  line L1366 (37.29, 34.0334) -> (37.0431, 34.0334) construction
  line L1367 (37.0431, 34.0334) -> (36.843, 33.8334) construction
  line L1368 (36.843, 33.8334) -> (36.843, 33.5866) construction
  spline S418 degree 3 poles (36.843, 33.5866) (36.843, 33.3398) (37.0431, 33.1395) (37.29, 33.1395) knots 0 0 0 0 1 1 1 1
  line L1369 (36.843, 33.5866) -> (36.843, 33.3398) construction
  line L1370 (36.843, 33.3398) -> (37.0431, 33.1395) construction
  line L1371 (37.0431, 33.1395) -> (37.29, 33.1395) construction
  spline S419 degree 3 poles (37.29, 33.1395) (37.5369, 33.1395) (37.737, 33.3398) (37.737, 33.5866) knots 0 0 0 0 1 1 1 1
  line L1372 (37.29, 33.1395) -> (37.5369, 33.1395) construction
  line L1373 (37.5369, 33.1395) -> (37.737, 33.3398) construction
  line L1374 (37.737, 33.3398) -> (37.737, 33.5866) construction
  spline S420 degree 3 poles (40.2911, 33.5866) (40.2911, 33.8334) (40.091, 34.0334) (39.8441, 34.0334) knots 0 0 0 0 1 1 1 1
  line L1375 (40.2911, 33.5866) -> (40.2911, 33.8334) construction
  line L1376 (40.2911, 33.8334) -> (40.091, 34.0334) construction
  line L1377 (40.091, 34.0334) -> (39.8441, 34.0334) construction
  spline S421 degree 3 poles (39.8441, 34.0334) (39.5972, 34.0334) (39.3971, 33.8334) (39.3971, 33.5866) knots 0 0 0 0 1 1 1 1
  line L1378 (39.8441, 34.0334) -> (39.5972, 34.0334) construction
  line L1379 (39.5972, 34.0334) -> (39.3971, 33.8334) construction
  line L1380 (39.3971, 33.8334) -> (39.3971, 33.5866) construction
  spline S422 degree 3 poles (39.3971, 33.5866) (39.3971, 33.3398) (39.5972, 33.1395) (39.8441, 33.1395) knots 0 0 0 0 1 1 1 1
  line L1381 (39.3971, 33.5866) -> (39.3971, 33.3398) construction
  line L1382 (39.3971, 33.3398) -> (39.5972, 33.1395) construction
  line L1383 (39.5972, 33.1395) -> (39.8441, 33.1395) construction
  spline S423 degree 3 poles (39.8441, 33.1395) (40.091, 33.1395) (40.2911, 33.3398) (40.2911, 33.5866) knots 0 0 0 0 1 1 1 1
  line L1384 (39.8441, 33.1395) -> (40.091, 33.1395) construction
  line L1385 (40.091, 33.1395) -> (40.2911, 33.3398) construction
  line L1386 (40.2911, 33.3398) -> (40.2911, 33.5866) construction
  spline S424 degree 3 poles (42.8452, 33.5866) (42.8452, 33.8334) (42.6451, 34.0334) (42.3982, 34.0334) knots 0 0 0 0 1 1 1 1
  line L1387 (42.8452, 33.5866) -> (42.8452, 33.8334) construction
  line L1388 (42.8452, 33.8334) -> (42.6451, 34.0334) construction
  line L1389 (42.6451, 34.0334) -> (42.3982, 34.0334) construction
  spline S425 degree 3 poles (42.3982, 34.0334) (42.1513, 34.0334) (41.9512, 33.8334) (41.9512, 33.5866) knots 0 0 0 0 1 1 1 1
  line L1390 (42.3982, 34.0334) -> (42.1513, 34.0334) construction
  line L1391 (42.1513, 34.0334) -> (41.9512, 33.8334) construction
  line L1392 (41.9512, 33.8334) -> (41.9512, 33.5866) construction
  spline S426 degree 3 poles (41.9512, 33.5866) (41.9512, 33.3398) (42.1513, 33.1395) (42.3982, 33.1395) knots 0 0 0 0 1 1 1 1
  line L1393 (41.9512, 33.5866) -> (41.9512, 33.3398) construction
  line L1394 (41.9512, 33.3398) -> (42.1513, 33.1395) construction
  line L1395 (42.1513, 33.1395) -> (42.3982, 33.1395) construction
  spline S427 degree 3 poles (42.3982, 33.1395) (42.6451, 33.1395) (42.8452, 33.3398) (42.8452, 33.5866) knots 0 0 0 0 1 1 1 1
  line L1396 (42.3982, 33.1395) -> (42.6451, 33.1395) construction
  line L1397 (42.6451, 33.1395) -> (42.8452, 33.3398) construction
  line L1398 (42.8452, 33.3398) -> (42.8452, 33.5866) construction
  spline S428 degree 3 poles (45.3993, 33.5866) (45.3993, 33.8334) (45.1992, 34.0334) (44.9523, 34.0334) knots 0 0 0 0 1 1 1 1
  line L1399 (45.3993, 33.5866) -> (45.3993, 33.8334) construction
  line L1400 (45.3993, 33.8334) -> (45.1992, 34.0334) construction
  line L1401 (45.1992, 34.0334) -> (44.9523, 34.0334) construction
  spline S429 degree 3 poles (44.9523, 34.0334) (44.7054, 34.0334) (44.5054, 33.8334) (44.5054, 33.5866) knots 0 0 0 0 1 1 1 1
  line L1402 (44.9523, 34.0334) -> (44.7054, 34.0334) construction
  line L1403 (44.7054, 34.0334) -> (44.5054, 33.8334) construction
  line L1404 (44.5054, 33.8334) -> (44.5054, 33.5866) construction
  spline S430 degree 3 poles (44.5054, 33.5866) (44.5054, 33.3398) (44.7054, 33.1395) (44.9523, 33.1395) knots 0 0 0 0 1 1 1 1
  line L1405 (44.5054, 33.5866) -> (44.5054, 33.3398) construction
  line L1406 (44.5054, 33.3398) -> (44.7054, 33.1395) construction
  line L1407 (44.7054, 33.1395) -> (44.9523, 33.1395) construction
  spline S431 degree 3 poles (44.9523, 33.1395) (45.1992, 33.1395) (45.3993, 33.3398) (45.3993, 33.5866) knots 0 0 0 0 1 1 1 1
  line L1408 (44.9523, 33.1395) -> (45.1992, 33.1395) construction
  line L1409 (45.1992, 33.1395) -> (45.3993, 33.3398) construction
  line L1410 (45.3993, 33.3398) -> (45.3993, 33.5866) construction
  spline S432 degree 3 poles (33.9058, 0.3832) (33.9058, 0.6299) (33.7056, 0.83) (33.4588, 0.83) knots 0 0 0 0 1 1 1 1
  line L1411 (33.9058, 0.3832) -> (33.9058, 0.6299) construction
  line L1412 (33.9058, 0.6299) -> (33.7056, 0.83) construction
  line L1413 (33.7056, 0.83) -> (33.4588, 0.83) construction
  spline S433 degree 3 poles (33.4588, 0.83) (33.212, 0.83) (33.0119, 0.6299) (33.0119, 0.3832) knots 0 0 0 0 1 1 1 1
  line L1414 (33.4588, 0.83) -> (33.212, 0.83) construction
  line L1415 (33.212, 0.83) -> (33.0119, 0.6299) construction
  line L1416 (33.0119, 0.6299) -> (33.0119, 0.3832) construction
  spline S434 degree 3 poles (33.0119, 0.3832) (33.0119, 0.1364) (33.212, -0.0639) (33.4588, -0.0639) knots 0 0 0 0 1 1 1 1
  line L1417 (33.0119, 0.3832) -> (33.0119, 0.1364) construction
  line L1418 (33.0119, 0.1364) -> (33.212, -0.0639) construction
  line L1419 (33.212, -0.0639) -> (33.4588, -0.0639) construction
  spline S435 degree 3 poles (33.4588, -0.0639) (33.7056, -0.0639) (33.9058, 0.1364) (33.9058, 0.3832) knots 0 0 0 0 1 1 1 1
  line L1420 (33.4588, -0.0639) -> (33.7056, -0.0639) construction
  line L1421 (33.7056, -0.0639) -> (33.9058, 0.1364) construction
  line L1422 (33.9058, 0.1364) -> (33.9058, 0.3832) construction
  spline S436 degree 3 poles (31.3517, 0.3832) (31.3517, 0.6299) (31.1515, 0.83) (30.9047, 0.83) knots 0 0 0 0 1 1 1 1
  line L1423 (31.3517, 0.3832) -> (31.3517, 0.6299) construction
  line L1424 (31.3517, 0.6299) -> (31.1515, 0.83) construction
  line L1425 (31.1515, 0.83) -> (30.9047, 0.83) construction
  spline S437 degree 3 poles (30.9047, 0.83) (30.6579, 0.83) (30.4578, 0.6299) (30.4578, 0.3832) knots 0 0 0 0 1 1 1 1
  line L1426 (30.9047, 0.83) -> (30.6579, 0.83) construction
  line L1427 (30.6579, 0.83) -> (30.4578, 0.6299) construction
  line L1428 (30.4578, 0.6299) -> (30.4578, 0.3832) construction
  spline S438 degree 3 poles (30.4578, 0.3832) (30.4578, 0.1364) (30.6579, -0.0639) (30.9047, -0.0639) knots 0 0 0 0 1 1 1 1
  line L1429 (30.4578, 0.3832) -> (30.4578, 0.1364) construction
  line L1430 (30.4578, 0.1364) -> (30.6579, -0.0639) construction
  line L1431 (30.6579, -0.0639) -> (30.9047, -0.0639) construction
  spline S439 degree 3 poles (30.9047, -0.0639) (31.1515, -0.0639) (31.3517, 0.1364) (31.3517, 0.3832) knots 0 0 0 0 1 1 1 1
  line L1432 (30.9047, -0.0639) -> (31.1515, -0.0639) construction
  line L1433 (31.1515, -0.0639) -> (31.3517, 0.1364) construction
  line L1434 (31.3517, 0.1364) -> (31.3517, 0.3832) construction
  spline S440 degree 3 poles (28.7976, 0.3832) (28.7976, 0.6299) (28.5974, 0.83) (28.3506, 0.83) knots 0 0 0 0 1 1 1 1
  line L1435 (28.7976, 0.3832) -> (28.7976, 0.6299) construction
  line L1436 (28.7976, 0.6299) -> (28.5974, 0.83) construction
  line L1437 (28.5974, 0.83) -> (28.3506, 0.83) construction
  spline S441 degree 3 poles (28.3506, 0.83) (28.1038, 0.83) (27.9037, 0.6299) (27.9037, 0.3832) knots 0 0 0 0 1 1 1 1
  line L1438 (28.3506, 0.83) -> (28.1038, 0.83) construction
  line L1439 (28.1038, 0.83) -> (27.9037, 0.6299) construction
  line L1440 (27.9037, 0.6299) -> (27.9037, 0.3832) construction
  spline S442 degree 3 poles (27.9037, 0.3832) (27.9037, 0.1364) (28.1038, -0.0639) (28.3506, -0.0639) knots 0 0 0 0 1 1 1 1
  line L1441 (27.9037, 0.3832) -> (27.9037, 0.1364) construction
  line L1442 (27.9037, 0.1364) -> (28.1038, -0.0639) construction
  line L1443 (28.1038, -0.0639) -> (28.3506, -0.0639) construction
  spline S443 degree 3 poles (28.3506, -0.0639) (28.5974, -0.0639) (28.7976, 0.1364) (28.7976, 0.3832) knots 0 0 0 0 1 1 1 1
  line L1444 (28.3506, -0.0639) -> (28.5974, -0.0639) construction
  line L1445 (28.5974, -0.0639) -> (28.7976, 0.1364) construction
  line L1446 (28.7976, 0.1364) -> (28.7976, 0.3832) construction
  spline S444 degree 3 poles (42.8452, 0.3832) (42.8452, 0.6299) (42.6451, 0.83) (42.3982, 0.83) knots 0 0 0 0 1 1 1 1
  line L1447 (42.8452, 0.3832) -> (42.8452, 0.6299) construction
  line L1448 (42.8452, 0.6299) -> (42.6451, 0.83) construction
  line L1449 (42.6451, 0.83) -> (42.3982, 0.83) construction
  spline S445 degree 3 poles (42.3982, 0.83) (42.1513, 0.83) (41.9512, 0.6299) (41.9512, 0.3832) knots 0 0 0 0 1 1 1 1
  line L1450 (42.3982, 0.83) -> (42.1513, 0.83) construction
  line L1451 (42.1513, 0.83) -> (41.9512, 0.6299) construction
  line L1452 (41.9512, 0.6299) -> (41.9512, 0.3832) construction
  spline S446 degree 3 poles (41.9512, 0.3832) (41.9512, 0.1364) (42.1513, -0.0639) (42.3982, -0.0639) knots 0 0 0 0 1 1 1 1
  line L1453 (41.9512, 0.3832) -> (41.9512, 0.1364) construction
  line L1454 (41.9512, 0.1364) -> (42.1513, -0.0639) construction
  line L1455 (42.1513, -0.0639) -> (42.3982, -0.0639) construction
  spline S447 degree 3 poles (42.3982, -0.0639) (42.6451, -0.0639) (42.8452, 0.1364) (42.8452, 0.3832) knots 0 0 0 0 1 1 1 1
  line L1456 (42.3982, -0.0639) -> (42.6451, -0.0639) construction